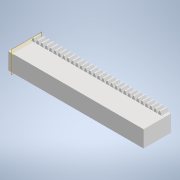
# Autodesk Inventor part: Rack gear m10 Z30
Saved by Autodesk Inventor 2022 (Build 260153000, 153)
## iProperties
Created: 2022-01-08
Part Number: Rack gear m10 Z30
Material: Generico
Document SubType Name: Modeling
Designer: Elia
Density: 1 g/cm^3
Appearance: Default
Author: Elia
Autodesk Inventor part; units mm, degrees
ref_plane "XZ Plane" through (0, 0, 0) normal (0, 1, 0) x (-1, 0, 0)
ref_plane "XY Plane" through (0, 0, 0) normal (0, 0, 1) x (1, 0, 0)
sketch "Schizzo5" plane through (0, 0, 0) normal (0, 0, 1) x (1, 0, 0)
  line L0 (-30, 0) -> (945, 0)
  line L1 (945, 0) -> (945, -120)
  line L2 (945, -120) -> (-30, -120)
  line L3 (-30, -120) -> (-30, 0)
  point P0 (0, 0)
  dimension "d16" = 120
  dimension "d17" = 975
  dimension "d18" = 30
  constraints: 8 end point, 2 parallel, 1 horizontal, 1 perpendicular
  measures "d16" distance of L2.end L0.start
  measures "d17" distance of L1.end L2.end
  measures "d18" distance of point (0, 0) L0.start
extrude "Estrusione3" add sketch "Schizzo5" along normal blind 175.35 and the other way blind 21.25
sketch "Schizzo6" plane through (0, 0, 0) normal (0, 0, 1) x (1, 0, 0)
  line L0 (-30, -120) -> (-30, 0) projected
  line L1 (-30, 0) -> (945, 0) projected
  line L2 (945, 0) -> (945, -120) projected
  line L3 (945, -120) -> (-30, -120) projected
  line L4 (0, 0) -> (0, 20.5559) construction
  line L5 (-4.2143, 22.5) -> (4.2143, 22.5)
  line L6 (4.2143, 22.5) -> (12.4036, 0)
  line L7 (945, 0) -> (-30, 0) projected
  line L8 (-4.2143, 22.5) -> (-12.4036, 0)
  line L9 (-7.854, 12.5) -> (7.854, 12.5) construction
  dimension "d21" = 40
  dimension "d22" = 22.5
  dimension "d23" = 10
  dimension "d24" = 15.708
  constraints: 10 end point, 4 point on line, 2 horizontal, 1 vertical, 1 other
  measures "d21" angle of L6 L8
  measures "d22" distance between parallel lines of L1 L5
  measures "d23" distance between parallel lines of L5 L9
  measures "d24" distance of L9.start L9.end
extrude "Estrusione4" add sketch "Schizzo6" along normal mid plane 52.5 contours L8 L5 L6 L1
fillet "Raccordo2" radius 3.8 2 edges at (12.4036, 0, 2.5) (-12.4036, 0, 2.5)
pattern_linear "Serie rettangolare2" count 30 spacing 31.4159 along (1, 0, 0) of "Estrusione4", "Raccordo2"
ref_plane "Piano di lavoro3" through (-4.2143, 12.5, 26.25) normal (0, 1, 0) x (1, 0, 0)
sketch "Schizzo7" plane through (0, 0, 175.35) normal (0, 0, 1) x (1, 0, 0)
  point P0 (0, 0)
